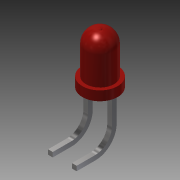
# Autodesk Inventor part: led
Saved by Autodesk Inventor 2014 SP1 (Build 180222100, 222)
## iProperties
Created: 2014-04-13
Part Number: led
Material: Generic
Document SubType Name: Modeling
Designer: Tyler
Density: 1 g/cm^3
Appearance: Orange-Red
Author: Tyler
Autodesk Inventor part; units mm, degrees
ref_plane "YZ Plane" through (0, 0, 0) normal (1, 0, 0) x (0, 1, 0)
ref_plane "XZ Plane" through (0, 0, 0) normal (0, 1, 0) x (-1, 0, 0)
ref_plane "XY Plane" through (0, 0, 0) normal (0, 0, 1) x (1, 0, 0)
sketch "Sketch1" plane through (0, 0, 0) normal (0, 0, 1) x (1, 0, 0)
  circle A0 centre (0, 0) radius 1.5
  dimension "d0" = 3
  constraints: 1 centre point, 1 coincident
  measures "d0" diameter of A0
extrude "Extrusion1" add sketch "Sketch1" along normal blind 4.49
fillet "Fillet1" radius 1.5 1 edges at (-1.5, 0, 4.49)
sketch "Sketch2" plane through (0, 0, 0) normal (0, 0, -1) x (-1, 0, 0)
  circle A0 centre (0, 0) radius 1.5 projected
  circle A1 centre (0, 0) radius 1.875
  dimension "d4" = 3.75
  constraints: 1 centre point, 1 coincident
  measures "d4" diameter of A1
extrude "Extrusion2" add sketch "Sketch2" along normal blind 1 contours A0 | A1
sketch "Sketch3" plane through (0, 0, -1) normal (0, 0, -1) x (-1, 0, 0)
  circle A0 centre (0, 0) radius 1.875 projected
  line L0 (-1.52, 0.25) -> (-1.02, 0.25)
  line L1 (-1.02, 0.25) -> (-1.02, -0.25)
  line L2 (-1.02, -0.25) -> (-1.52, -0.25)
  line L3 (-1.52, -0.25) -> (-1.52, 0.25)
  line L4 (1.02, 0.25) -> (1.52, 0.25)
  line L5 (1.52, 0.25) -> (1.52, -0.25)
  line L6 (1.52, -0.25) -> (1.02, -0.25)
  line L7 (1.02, -0.25) -> (1.02, 0.25)
  dimension "d7" = 0.5
  dimension "d8" = 0.5
  dimension "d9" = 0.5
  dimension "d10" = 0.5
  dimension "d11" = 0.25
  dimension "d12" = 0.25
  dimension "d13" = 1.02
  dimension "d14" = 1.02
  constraints: 16 end point, 4 parallel, 2 horizontal, 2 perpendicular
  measures "d7" distance of L0.start L0.end
  measures "d8" distance of L2.end L0.start
  measures "d9" distance of L4.end L5.end
  measures "d10" distance of L4.start L4.end
  measures "d11" distance from line of A0.centre L4
  measures "d12" distance from line of A0.centre L0
  measures "d13" distance from line of A0.centre L1
  measures "d14" distance from line of A0.centre L7
sketch "Sketch4" plane through (0, 0, 0) normal (1, 0, 0) x (0, 1, 0)
  line L0 (0, -0.5) -> (0, -3.75)
  line L1 (-2, -5.75) -> (-4, -5.75)
  line L2 (-1.875, -1) -> (1.875, -1) projected
  arc A0 (-2, -5.75) -> (0, -3.75) centre (-2, -3.75) ccw
  line L3 (1.875, 0) -> (-1.875, 0) projected
  point P0 (0, 0)
  point P1 (0, -5.75)
  dimension "d16" = 4
  dimension "d17" = 5.25
  dimension "d18" = 2
  dimension "d19" = 1.875
  dimension "d21" = 0.5
  constraints: 4 end point, 2 point on circle, 2 point on line, 2 tangent, 1 centre point, 1 perpendicular, 1 vertical
  measures "d16" distance of point (0, -5.75) L1.end
  measures "d17" distance of L0.start point (0, -5.75)
  measures "d18" radius of A0
  measures "d19" distance from line of L2.end L0
  measures "d21" distance from line of L3 L0.start
sweep "Sweep1" add profiles "Sketch3" path "Sketch4" path curves L0 A0 L1 contours L0 L1 L2 L3 | L4 L5 L6 L7
body "Solid1"
